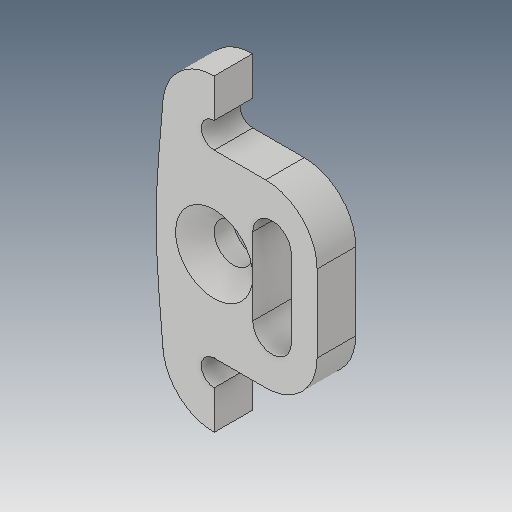
# Autodesk Inventor part: ShaftBase2
Saved by Autodesk Inventor 2019.4 (Build 234330000, 330)
## iProperties
Created: 2019-06-11
Part Number: ShaftBase2
Material: Generic
Document SubType Name: Modeling
Designer: AzLIer
Density: 1 g/cm^3
Appearance: Default
Mass: 0.478074 g
Surface Area: 6.17696 cm^2
Volume: 0.478074 cm^3
Author: AzLIer
Autodesk Inventor part; units mm, degrees
note: some values were not read from the file. Chosen so that the rebuilt part matches the saved one: second side of "押し出し1".
ref_plane "YZ Plane" through (0, 0, 0) normal (1, 0, 0) x (0, 1, 0)
ref_plane "XZ Plane" through (0, 0, 0) normal (0, 1, 0) x (-1, 0, 0)
ref_plane "XY Plane" through (0, 0, 0) normal (0, 0, 1) x (1, 0, 0)
sketch "スケッチ1" plane through (0, 0, 0) normal (0, 0, 1) x (1, 0, 0)
  line L0 (-4, -7) -> (0, -7)
  line L1 (4, -3) -> (4, 0)
  arc A0 (-4, -7) -> (-4, -9) centre (-4, -8) ccw
  line L2 (-4, -9) -> (-4, -12)
  arc A1 (-5.5, 0) -> (-2.5, 0) centre (-4, 0) ccw
  arc A2 (-7.9856, -8.3391) -> (-4, -12) centre (-4, -8) ccw
  line L3 (-7.9856, -8.3391) -> (-8.3056, -4.5778)
  line L4 (-8.5, 0) -> (-5.5, 0)
  line L5 (-1, 0) -> (-1, -3)
  line L6 (2, -3) -> (2, 0)
  line L7 (-2.5, 0) -> (-1, 0)
  line L8 (2, 0) -> (4, 0)
  arc A3 (-1, -3) -> (2, -3) centre (0.5, -3) ccw
  circle A4 centre (-4, 0) radius 5 construction
  line L9 (-9, 0) -> (-9, -7) construction
  arc A5 (-8.5, 0) -> (-8.3056, -4.5778) centre (45.5, 0) ccw
  circle A6 centre (-4, 0) radius 3 construction
  arc A7 (0, -7) -> (4, -3) centre (0, -3) ccw
  point P0 (0, 0)
  point P1 (0, 0)
  point P2 (0, 0)
  dimension "d14" = 10
  dimension "d17" = 6
  dimension "d3" = 1
  dimension "d4" = 3
  dimension "d6" = 3
  dimension "d8" = 4
  dimension "d11" = 3
  dimension "d13" = 2
  dimension "d15" = 5
  dimension "d16" = 54
  dimension "d31" = 4
  dimension "d32" = 7
  dimension "d41" = 4
  dimension "d42" = 4
  dimension "d43" = 4
  dimension "d46" = 1.5
  dimension "d47" = 3
  dimension "d48" = 3
  dimension "d53" = 0
  constraints: 21 end point, 12 point on circle, 6 centre point, 5 tangent, 5 vertical, 4 horizontal alignment, 4 point on line, 3 horizontal, 2 coincident, 2 parallel, 2 vertical alignment, 1 line through centre, 4 other
  measures "d3" radius of A0
  measures "d4" diameter of A1
  measures "d6" distance of L2.start L2.end
  measures "d8" radius of A2
  measures "d11" distance of L6.start L5.end
  measures "d13" distance between parallel lines of L1 L6
  measures "d15" distance between parallel lines of L2 L9
  measures "d16" radius of A5
  measures "d31" radius of A7
  measures "d32" distance between parallel lines of L0 L8
  measures "d41" distance from line of point (0, 0) L1
  measures "d42" distance from line of point (0, 0) L1
  measures "d43" distance from line of point (0, 0) L1
  measures "d46" radius of A3
  measures "d47" distance from line of L8 A3.centre
  measures "d48" distance of L4.start L4.end
  measures "d53" distance from line of point (0, 0) L8
extrude "押し出し1" add sketch "スケッチ1" along normal blind 3
mirror "ミラー1" about plane through (-1, 0, 0) normal (0, 1, 0) of "押し出し1"
chamfer "面取り1" distance 1.5 angle 45 1 edges at (-4, -1.5, 3)
